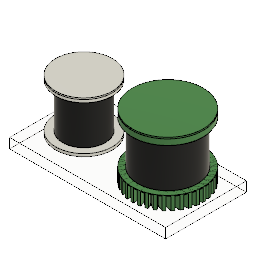
Booster (Autodesk Fusion 360 design; units mm, degrees)
Autodesk Fusion 360 part; units mm, degrees
note: some values were not read from the file. Set by a fixed rule: which sketch regions a step uses.
sketch "Esboço1" plane through (0, 0, 0) normal (0, 0, 1) x (1, 0, 0)
  line L0 (0, 0) -> (110, 0)
  line L1 (110, 0) -> (110, 57)
  line L2 (110, 57) -> (0, 57)
  line L3 (0, 57) -> (0, 0)
  dimension "d1" = 110
  dimension "d2" = 57
  constraint horizontal L0
  constraint vertical L1
  constraint horizontal L2
  constraint vertical L3
  constraint coincident L0.start L3.end
  measures "d1" distance of L1.end L2.end
  measures "d2" distance of L0.start L2.end
extrude "Extrusão1" add sketch "Esboço1" along normal blind 7 makes body 1
sketch "Esboço2" plane through (0, 0, 7) normal (0, 0, 1) x (-1, 0, 0)
  line L0 (0, -57) -> (0, 0)
  line L1 (0, 0) -> (-110, 0)
  line L2 (-110, 0) -> (-110, -57)
  line L3 (-110, -57) -> (0, -57)
  line L4 (-55, -57) -> (-55, 0) construction
  line L5 (0, -28.5) -> (-110, -28.5) construction
  circle A0 centre (-24, -28.5) radius 20
  circle A1 centre (-83, -28.5) radius 25
  circle A2 centre (-24, -28.5) radius 15
  circle A3 centre (-83, -28.5) radius 21
  dimension "d5" = 40
  dimension "d6" = 30
  dimension "d7" = 42
  dimension "d8" = 50
  dimension "d35" = 59
  dimension "d36" = 24
  constraint midpoint L3 L4.start
  constraint midpoint L1 L4.end
  constraint midpoint L0 L5.start
  constraint perpendicular L2 L5
  constraint midpoint L2 L5.end
  constraint coincident L5 A0.centre
  constraint coincident L5 A1.centre
  constraint concentric A0 A2
  constraint concentric A1 A3
  measures "d5" diameter of A0
  measures "d6" diameter of A2
  measures "d7" diameter of A3
  measures "d8" diameter of A1
  measures "d35" distance of A0.centre A1.centre
  measures "d36" distance of L0 A0.centre
extrude "Extrusão2" add sketch "Esboço2" along normal blind 2 separate body contours A0 makes body 2
extrude "Extrusão3" add sketch "Esboço2" along normal blind 35 separate body contours A2 makes body 3
sketch "Esboço3" plane through (0, 0, 42) normal (0, 0, 1) x (-1, 0, 0)
  circle A0 centre (-24, -28.5) radius 15
  circle A1 centre (-24, -28.5) radius 20
  circle A2 centre (-24, -28.5) radius 15
  dimension "d13" = 40
  dimension "d14" = 30
  constraint concentric A0 A1
  constraint concentric A1 A2
  measures "d13" diameter of A1
  measures "d14" diameter of A2
extrude "Extrusão4" add sketch "Esboço3" against normal blind 2 separate body makes body 4
extrude "Extrusão5" add sketch "Esboço3" along normal blind 1 separate body contours A0 A2 | A1 makes body 5
extrude "Extrusão6" add sketch "Esboço2" along normal blind 9.5 separate body contours A1 makes body 6
extrude "Extrusão7" add sketch "Esboço2" along normal blind 44 separate body contours A3 makes body 7
sketch "Esboço4" plane through (0, 0, 51) normal (0, 0, 1) x (-1, 0, 0)
  circle A0 centre (-83, -28.5) radius 21
  circle A1 centre (-83, -28.5) radius 21
  circle A2 centre (-83, -28.5) radius 25
  dimension "d23" = 42
  dimension "d24" = 50
  constraint concentric A0 A1
  constraint concentric A1 A2
  measures "d23" diameter of A1
  measures "d24" diameter of A2
extrude "Extrusão8" add sketch "Esboço4" against normal blind 4 separate body makes body 8
extrude "Extrusão9" add sketch "Esboço4" along normal blind 1 separate body contours A0 A1 | A2 makes body 9
ref_plane "Plano de trabalho1" through (83, 28.5, 16) normal (0, 0, 1) x (-1, 0, 0)
sketch "Esboço5" plane through (0, 0, 16) normal (0, 0, 1) x (-1, 0, 0)
  line L0 (-104, -28.5) -> (-108, -28.5)
  line L1 (-108, -28.5) -> (-103.8507, -26)
  line L2 (-107.8747, -26) -> (-103.8507, -26)
  line L3 (-107.8747, -26) -> (-108.6899, -27.8048)
  line L4 (-108, -28.5) -> (-108.6899, -27.8048)
  circle A0 centre (-83, -28.5) radius 21
  circle A1 centre (-83, -28.5) radius 25
  circle A2 centre (-83, -28.5) radius 21
  circle A3 centre (-83, -28.5) radius 25
  line L5 (0, -28.5) -> (-110, -28.5)
  point P0 (-83, -28.5)
  dimension "d29" = 2.5
  constraint horizontal L0
  constraint parallel L0 L2
  constraint concentric A0 A1
  constraint coincident P0 A0.centre
  constraint tangent A0 A2
  constraint tangent A1 A3
  constraint coincident L0.end A1
  constraint coincident L0.start A0
  constraint coincident L1.end A0
  constraint coincident L2.start A1
  constraint coincident L0.end L5
  measures "d29" vertical distance of L0.end L2.start
extrude "Extrusão10" cut sketch "Esboço5" against normal up to surface (9 mm away) contours L1 L2 A1 A3 | L3 L4 A1 A3 bodies 6
pattern_circular "Padrão circular1" count 35 over 360 about axis through (83, 28.5, 16.5) along (0, 0, -1) of "Extrusão10"
equation "d35 = d5 / 2 + d8 / 2 + 14 mm"
equation "d36 = d5 / 2 + 4 mm"
